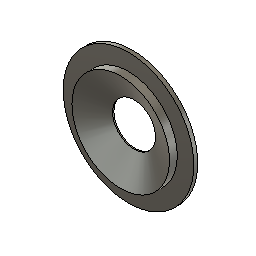
Anillo Inyector Pelton v3 (Autodesk Fusion 360 design; units mm, degrees)
Autodesk Fusion 360 part; units mm, degrees
note: some values were not read from the file. Set by a fixed rule: which sketch regions a step uses.
sketch "Sketch2" plane through (0, 0, 0) normal (0, 1, 0) x (1, 0, 0)
  line L0 (-480, 0) -> (-480, -30)
  line L1 (-670, -30) -> (-670, -70)
  line L2 (-220, 0) -> (-220, -12.7)
  line L3 (-500, -150.3) -> (-220, -12.7)
  line L4 (-480, 0) -> (-220, 0)
  line L5 (-480, -30) -> (-670, -30)
  line L6 (-670, -70) -> (-500, -70)
  line L7 (-500, -70) -> (-500, -150.3)
  dimension "d17" = 30
  dimension "d18" = 40
  dimension "d19" = 12.7
  dimension "d22" = 190
  dimension "d23" = 170
  dimension "d24" = 80.3
  constraint perpendicular L2 L4
  constraint perpendicular L0 L5
  constraint perpendicular L1 L6
  constraint perpendicular L6 L7
  measures "d17" distance of L0.start L0.end
  measures "d18" distance of L1.start L1.end
  measures "d19" distance of L2.start L2.end
  measures "d22" distance of L0.end L1.start
  measures "d23" distance of L1.end L6.end
  measures "d24" distance of L6.end L3.start
revolve "Revolve1" add sketch "Sketch2" angle 360 about axis through (0, 0, 1.75) along (0, 0, 1)
